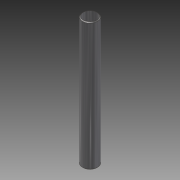
# Autodesk Inventor part: Rebuild Shooter NCDME075-0600 Body
Saved by Autodesk Inventor 2014 SP1 (Build 180222100, 222)
## iProperties
Created: 2013-12-19
Part Number: Rebuild Shooter NCDME075-0600 Body
Material: Stainless Steel
Document SubType Name: Modeling
Designer: Moses
Density: 8.08 g/cm^3
Appearance: Semi-Polished
Mass: 111.929 g
Surface Area: 242.406 cm^2
Volume: 13.8526 cm^3
Author: Moses
Autodesk Inventor part; units mm, degrees
ref_plane "YZ Plane" through (0, 0, 0) normal (1, 0, 0) x (0, 1, 0)
ref_plane "XZ Plane" through (0, 0, 0) normal (0, 1, 0) x (-1, 0, 0)
ref_plane "XY Plane" through (0, 0, 0) normal (0, 0, 1) x (1, 0, 0)
sketch "Sketch1" plane through (0, 0, 0) normal (1, 0, 0) x (0, 1, 0)
  line L0 (0, 0) -> (185.293, 0)
  line L1 (0, 10.922) -> (185.293, 10.922)
  line L2 (0, 10.922) -> (0, 9.779) construction
  line L3 (0, 9.779) -> (185.293, 9.779)
  line L4 (185.293, 9.779) -> (185.293, 10.922) construction
  line L5 (0, 9.779) -> (0, 0) construction
  line L6 (185.293, 9.779) -> (185.293, 0) construction
  line L7 (0, 9.779) -> (1.143, 10.922)
  line L8 (185.293, 9.779) -> (184.15, 10.922)
  line L9 (0, 9.779) -> (0, 8.89)
  line L10 (0, 8.89) -> (3.175, 8.89)
  line L11 (3.175, 8.89) -> (3.175, 9.779)
  dimension "d0" = 185.293
  dimension "d2" = 19.558
  dimension "d3" = 45
  dimension "d5" = 21.844
  dimension "d6" = 3.175
  dimension "d7" = 17.78
  constraints: 24 end point, 5 vertical, 4 horizontal, 4 point on line, 1 perpendicular
  measures "d0" distance of L0.start L0.end
  measures "d2" diameter of L3 L0
  measures "d3" angle of L4 L8
  measures "d5" diameter of L1.start L0
  measures "d6" distance of L9.end L10.end
  measures "d7" diameter of L9.end L0
revolve "Revolution1" add sketch "Sketch1" angle 360 about axis through (0, 0, 0) along (0, 1, 0)
body "Solid1"
